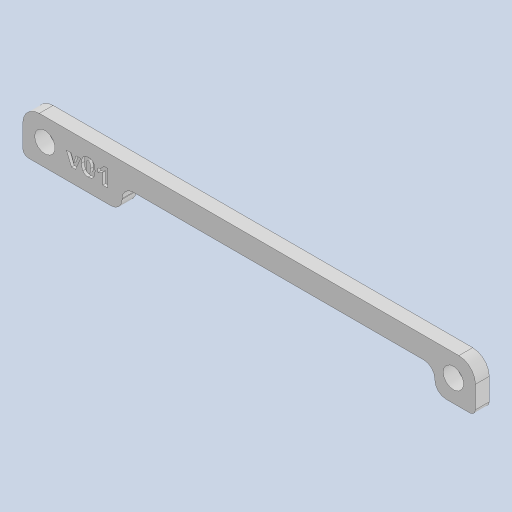
# Autodesk Inventor part: door_center_01
Saved by Autodesk Inventor 2024.4 (Build 284460030, 460C)
## iProperties
Created: 2026-07-13
Part Number: door_center_01
Material: Generic
Document SubType Name: Modeling
Designer: tooles01
Density: 1 g/cm^3
Appearance: Default
Author: tooles01
Autodesk Inventor part; units mm, degrees
ref_plane "YZ Plane" through (0, 0, 0) normal (1, 0, 0) x (0, 1, 0)
ref_plane "XZ Plane" through (0, 0, 0) normal (0, 1, 0) x (-1, 0, 0)
ref_plane "XY Plane" through (0, 0, 0) normal (0, 0, 1) x (1, 0, 0)
derived "door_front_01.ipt"
sketch "Sketch1: base" plane through (0, 0, 0) normal (0, 0, 1) x (1, 0, 0)
  line L0 (-41, 85) -> (41, 85)
  line L1 (41, 85) -> (41, 0)
  line L2 (41, 0) -> (-41, 0)
  line L3 (-41, 0) -> (-41, 85)
  circle A0 centre (0, 30) radius 16.25
  line L4 (-37, 81) -> (37, 81) construction
  line L5 (37, 81) -> (37, 4) construction
  line L6 (37, 4) -> (-37, 4) construction
  line L7 (-37, 4) -> (-37, 81) construction
  point P0 (0, 0)
  point P1 (0, 0)
  point P2 (0, 4)
sketch "Sketch5: PCB footprint" plane through (0, 0, 0) normal (0, 0, 1) x (1, 0, 0)
  line L0 (-0.5, 81) -> (34, 81)
  line L1 (34, 81) -> (34, 49)
  line L2 (34, 49) -> (-0.5, 49)
  line L3 (-0.5, 49) -> (-0.5, 81)
  circle A0 centre (2, 79) radius 1.5
  circle A1 centre (31.5, 79) radius 1.5
  circle A2 centre (2, 52) radius 1.5
  circle A3 centre (31.5, 52) radius 1.5
  line L4 (2, 79) -> (31.5, 79) construction
  line L5 (31.5, 79) -> (31.5, 52) construction
  line L6 (31.5, 52) -> (2, 52) construction
  line L7 (2, 52) -> (2, 79) construction
  circle A4 centre (0, 30) radius 17.75
  line L8 (41, 0) -> (41, 85)
  point P0 (0, 0)
  point P1 (16.75, 79)
  point P2 (16.75, 81)
sketch "Sketch: base" plane through (0, 0, 0) normal (0, 0, 1) x (1, 0, 0)
  line L0 (-41, 85) -> (41, 85) projected
  line L1 (-41, 0) -> (-41, 85) projected
  line L2 (41, 85) -> (41, 0) projected
  line L3 (-41, 77) -> (41, 77)
  line L4 (-23, 81.15) -> (33.65, 81.15)
  line L5 (33.65, 81.15) -> (33.65, 77)
  line L6 (-23, 77) -> (-23, 81.15)
  circle A0 centre (2, 79) radius 1.5 construction
  circle A1 centre (31.5, 79) radius 1.5 construction
  circle A2 centre (31.5, 79) radius 2.1 construction
  circle A3 centre (2, 79) radius 2.1 construction
  circle A4 centre (37, 81) radius 1.85 construction
  point P0 (0, 0)
  point P1 (-37, 81)
  dimension "d15" = 8
  dimension "d17" = 4.2
  dimension "d18" = 2.15
  dimension "d19" = 2.15
  dimension "d20" = 18
  dimension "d36" = 3.7
  dimension "d40" = 3.35
  constraints: 8 end point, 4 perpendicular, 4 point on line, 3 centre point, 3 coincident, 1 equal radius
  measures "d15" distance between parallel lines of L0 L3
  measures "d17" diameter of A2
  measures "d18" distance from line of L5 A1.centre
  measures "d19" distance from line of L4 A1.centre
  measures "d20" distance between parallel lines of L1 L6
  measures "d36" diameter of A4
  measures "d40" distance from line of L5 point (37, 81)
extrude "Ex1: base" add sketch "Sketch: base" against normal blind 2.5 contours L0 L2 L3 L5 L4 L6 L1
sketch "Sketch: text" plane through (0, 0, 0) normal (0, 0, 1) x (1, 0, 0)
  line L0 (-30.5, 82.5) -> (-27.5, 82.5) construction
  line L1 (-27.5, 82.5) -> (-27.5, 79.5) construction
  line L2 (-27.5, 79.5) -> (-30.5, 79.5) construction
  line L3 (-30.5, 79.5) -> (-30.5, 82.5) construction
  line L4 (-41, 85) -> (41, 85) construction
  line L5 (-41, 77) -> (41, 77) construction
  line L6 (-41, 85) -> (-41, 77) construction
  line L7 (-33.0727, 81.6742) -> (-32.2064, 81.6742)
  line L8 (-32.2064, 81.6742) -> (-31.782, 80.2969)
  line L9 (-31.782, 80.2969) -> (-31.346, 81.6742)
  line L10 (-31.346, 81.6742) -> (-30.5058, 81.6742)
  line L11 (-30.5058, 81.6742) -> (-31.4297, 79.5)
  line L12 (-31.4297, 79.5) -> (-32.1689, 79.5)
  line L13 (-32.1689, 79.5) -> (-33.0727, 81.6742)
  spline S0 degree 2 poles (-30.3441, 81.013) (-30.3441, 81.8677) (-29.7291, 82.552) (-29.0996, 82.552) knots 0 0 0 1 2 2 2
  spline S1 degree 2 poles (-29.0996, 82.552) (-28.7964, 82.552) (-28.4095, 82.4018) (-28.1641, 82.1622) (-28.0226, 81.8994) (-27.9793, 81.7233) knots 0 0 0 1 2 3 4 4 4
  spline S2 degree 2 poles (-27.9793, 81.7233) (-27.8956, 81.3884) (-27.8956, 81.0217) knots 0 0 0 1 1 1
  spline S3 degree 2 poles (-27.8956, 81.0217) (-27.8956, 80.2045) (-28.4471, 79.448) (-29.1227, 79.448) knots 0 0 0 1 2 2 2
  spline S4 degree 2 poles (-29.1227, 79.448) (-29.501, 79.448) (-29.9658, 79.6906) (-30.116, 79.9244) knots 0 0 0 1 2 2 2
  spline S5 degree 2 poles (-30.116, 79.9244) (-30.2228, 80.089) (-30.3441, 80.6636) (-30.3441, 81.013) knots 0 0 0 1 2 2 2
  spline S6 degree 2 poles (-29.5183, 81.0101) (-29.5183, 80.4355) (-29.3162, 80.0168) (-29.1256, 80.0168) knots 0 0 0 1 2 2 2
  spline S7 degree 2 poles (-29.1256, 80.0168) (-28.9986, 80.0168) (-28.8109, 80.1959) (-28.7243, 80.5799) (-28.7243, 80.987) knots 0 0 0 1 2 3 3 3
  spline S8 degree 2 poles (-28.7243, 80.987) (-28.7243, 81.5847) (-28.9264, 81.9976) (-29.1285, 81.9976) knots 0 0 0 1 2 2 2
  spline S9 degree 2 poles (-29.1285, 81.9976) (-29.3335, 81.9976) (-29.5183, 81.5789) (-29.5183, 81.0101) knots 0 0 0 1 2 2 2
  line L14 (-25.6578, 82.552) -> (-25.6578, 79.5)
  line L15 (-25.6578, 79.5) -> (-26.501, 79.5)
  line L16 (-26.501, 79.5) -> (-26.501, 81.501)
  spline S10 degree 2 poles (-26.501, 81.501) (-26.706, 81.345) (-27.0871, 81.1545) (-27.3758, 81.065) knots 0 0 0 1 2 2 2
  line L17 (-27.3758, 81.065) -> (-27.3758, 81.7493)
  spline S11 degree 2 poles (-27.3758, 81.7493) (-26.9514, 81.885) (-26.4808, 82.269) (-26.3479, 82.552) knots 0 0 0 1 2 2 2
  line L18 (-26.3479, 82.552) -> (-25.6578, 82.552)
  point P0 (0, 0)
  point P1 (-29, 82.5)
  point P2 (0, 85)
  point P3 (-41, 81)
  point P4 (-30.5, 81)
  dimension "d12" = 3
  dimension "d16" = 12
  constraints: 4 midpoint, 2 end point, 1 horizontal, 1 horizontal alignment, 1 perpendicular, 2 other
  measures "d12" distance of L0.start L0.end
  measures "d16" distance from line of point (-29, 82.5) L6
extrude "Ex2: text" cut sketch "Sketch: text" against normal blind 0.5
hole "Hole1: mounting (M3 thru holes)" at (37, 81, 0) at (-37, 81, 0) direction (0, 0, -1) diameter 3.7 end through all both
fillet "Fillet1" radius 3 2 edges at (-41, 85, -1.25) (41, 85, -1.25)
fillet "Fillet2" radius 2 4 edges at (-23, 81.15, -1.25) (33.65, 81.15, -1.25) (-23, 77, -1.25) (33.65, 77, -1.25)
fillet "Fillet3" radius 1 2 edges at (41, 77, -1.25) (-41, 77, -1.25)
equation "\"d17\" = d61"
equation "\"d19\" = d18"
equation "\"d61\" = 4.2"
body "Solid1"
